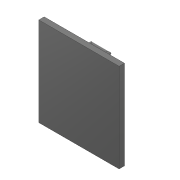
# Autodesk Inventor part: DeckelMess
Saved by Autodesk Inventor 2020 (Build 240168000, 168)
## iProperties
Created: 2022-01-25
Part Number: DeckelMess
Material: Acetalharz, Schwarz
Document SubType Name: Modeling
Designer: Julian Uhl
Density: 1.425 g/cm^3
Appearance: Glatt - Schwarz
Author: Julian Uhl
Autodesk Inventor part; units mm, degrees
ref_plane "YZ Plane" through (0, 0, 0) normal (1, 0, 0) x (0, 1, 0)
ref_plane "XZ Plane" through (0, 0, 0) normal (0, 1, 0) x (-1, 0, 0)
ref_plane "XY Plane" through (0, 0, 0) normal (0, 0, 1) x (1, 0, 0)
sketch "Skizze1" plane through (0, 0, 0) normal (0, 0, 1) x (1, 0, 0)
  line L0 (-24, 0) -> (144, 0) projected
  line L1 (0, -27.6) -> (0, 165.6) projected
  line L2 (0, 0) -> (120, 0)
  line L3 (120, 0) -> (120, 138)
  line L4 (120, 138) -> (0, 138)
  line L5 (0, 138) -> (0, 0)
  point P0 (0, 138)
  dimension "d0" = 120
  dimension "d1" = 138
  constraints: 8 end point, 2 parallel, 1 horizontal, 1 perpendicular
  measures "d0" distance between parallel lines of L3 L1
  measures "d1" distance between parallel lines of L0 L4
extrude "Extrusion1" add sketch "Skizze1" along normal blind 8
sketch "Skizze2" plane through (0, 0, 0) normal (0, 0, -1) x (-1, 0, 0)
  line L0 (-75, 118) -> (-70, 118)
  line L1 (-70, 118) -> (-70, 113)
  line L2 (-70, 113) -> (-75, 113)
  line L3 (-75, 113) -> (-75, 118)
  line L4 (-50, 118) -> (-45, 118)
  line L5 (-45, 118) -> (-45, 113)
  line L6 (-45, 113) -> (-50, 113)
  line L7 (-50, 113) -> (-50, 118)
  line L8 (0, 138) -> (0, 0) projected
  line L9 (-120, 0) -> (-120, 138) projected
  line L10 (-120, 138) -> (0, 138) projected
  dimension "d4" = 5
  dimension "d5" = 5
  dimension "d6" = 5
  dimension "d7" = 5
  dimension "d8" = 45
  dimension "d9" = 45
  dimension "d10" = 20
  dimension "d11" = 20
  constraints: 16 end point, 4 parallel, 2 horizontal, 2 perpendicular
  measures "d4" distance between parallel lines of L6 L4
  measures "d5" distance between parallel lines of L5 L7
  measures "d6" distance from line of L2 L0.start
  measures "d7" distance between parallel lines of L3 L1
  measures "d8" distance between parallel lines of L8 L5
  measures "d9" distance between parallel lines of L9 L3
  measures "d10" distance between parallel lines of L10 L0
  measures "d11" distance between parallel lines of L10 L4
extrude "Extrusion2" add sketch "Skizze2" along normal blind 20
sketch "Skizze3" plane through (0, 0, -20) normal (0, 0, -1) x (-1, 0, 0)
  line L0 (-70, 118) -> (-75, 118) projected
  line L1 (-70, 113) -> (-70, 118) projected
  line L2 (-75, 118) -> (-70, 118)
  line L3 (-70, 118) -> (-70, 113)
  line L4 (-70, 113) -> (-75, 113)
  line L5 (-75, 113) -> (-75, 118)
  point P0 (0, 0)
  constraints: 8 end point, 2 parallel, 1 horizontal, 1 perpendicular
extrude "Extrusion3" add sketch "Skizze3" along normal blind 5
sketch "Skizze4" plane through (70, 113, 0) normal (-1, 0, 0) x (0, 0, 1)
  line L0 (0, 5) -> (-25, 5) projected
  line L1 (-20, 5) -> (-20, 0) projected
  line L2 (-25, 5) -> (-20, 5)
  line L3 (-20, 5) -> (-20, 0)
  line L4 (-20, 0) -> (-25, 0)
  line L5 (-25, 0) -> (-25, 5)
  point P0 (0, -113)
  constraints: 8 end point, 2 parallel, 1 horizontal, 1 perpendicular
extrude "Extrusion4" add sketch "Skizze4" along normal blind 25
fillet "Rundung1" radius 2.5 12 edges at (70, 113, -10) (75, 113, -12.5) (60, 113, -20) (60, 113, -25) (50, 113, -10) (45, 113, -12.5) (60, 118, -25) (70, 118, -10) (75, 118, -12.5) (60, 118, -20) (45, 118, -12.5) (50, 118, -10)
sketch "Skizze7" plane through (0, 0, 0) normal (0, 0, -1) x (-1, 0, 0)
  point P0 (0, 0)
sketch "Skizze8" plane through (0, 0, 0) normal (0, 0, -1) x (-1, 0, 0)
  line L0 (-120, 0) -> (-120, 138) projected
  line L1 (0, 138) -> (0, 0) projected
  line L2 (-120, 5) -> (0, 5)
  line L3 (0, 5) -> (0, 0)
  line L4 (0, 0) -> (-120, 0)
  line L5 (-120, 0) -> (-120, 5)
  point P0 (0, 5)
  dimension "d25" = 5
  constraints: 8 end point, 2 parallel, 1 horizontal, 1 perpendicular, 1 point on line
  measures "d25" distance between parallel lines of L4 L2
extrude "Extrusion7" cut sketch "Skizze8" against normal blind 10
